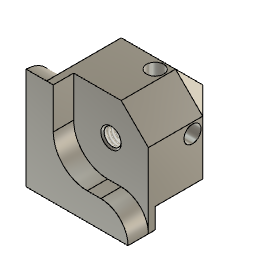
cornerstone-a (Autodesk Fusion 360 design; units mm, degrees)
Autodesk Fusion 360 part; units mm, degrees
sketch "Sketch1" plane through (0, 0, 0) normal (0, 0, 1) x (1, 0, 0)
  line L0 (0, 0) -> (15, 0)
  line L1 (15, 0) -> (15, 15)
  line L2 (15, 15) -> (0, 15)
  line L3 (0, 15) -> (0, 0)
  dimension "d5" = 15
  dimension "d6" = 15
  constraint horizontal L0
  constraint vertical L1
  constraint horizontal L2
  constraint vertical L3
  constraint coincident L0.start L3.end
  measures "d5" distance of L0.start L0.end
  measures "d6" distance of L0.start L2.end
extrude "Extrude1" add sketch "Sketch1" along normal blind 15
sketch "Sketch2" plane through (0, 0, 0) normal (0, -1, 0) x (1, 0, 0)
  line L0 (0, 0) -> (15, 0)
  line L1 (15, 0) -> (15, 15)
  line L2 (15, 15) -> (0, 15)
  line L3 (0, 15) -> (0, 0)
  line L4 (4, 4) -> (15, 4)
  line L5 (15, 4) -> (15, 15)
  line L6 (15, 15) -> (4, 15)
  line L7 (4, 15) -> (4, 4)
  point P0 (4, 4)
  dimension "d9" = 4
  dimension "d10" = 4
  constraint horizontal L4
  constraint vertical L5
  constraint horizontal L6
  constraint vertical L7
  constraint coincident L1.end L2.start
  constraint coincident P0 L4.start
  measures "d9" distance of L3 P0
  measures "d10" distance of L0 P0
extrude "Extrude2" cut sketch "Sketch2" against normal blind 3 contours L1 L2 L4 L5 L6 L7
sketch "Sketch3" plane through (0, 0, 0) normal (-1, 0, 0) x (0, -1, 0)
  line L0 (-15, 0) -> (0, 0)
  line L1 (0, 0) -> (0, 15)
  line L2 (0, 15) -> (-15, 15)
  line L3 (-15, 15) -> (-15, 0)
  line L4 (-4, 4) -> (-15, 4)
  line L5 (-15, 4) -> (-15, 15)
  line L6 (-15, 15) -> (-4, 15)
  line L7 (-4, 15) -> (-4, 4)
  point P0 (-4, 4)
  dimension "d14" = 4
  dimension "d15" = 4
  constraint horizontal L4
  constraint vertical L5
  constraint horizontal L6
  constraint vertical L7
  constraint coincident L2.end L3.start
  constraint coincident P0 L4.start
  measures "d14" distance of L1 P0
  measures "d15" distance of L0 P0
extrude "Extrude3" cut sketch "Sketch3" against normal blind 3 contours L2 L3 L4 L5 L6 L7
sketch "Sketch4" plane through (0, 0, 0) normal (0, 0, -1) x (1, 0, 0)
  line L0 (0, 0) -> (0, -15)
  line L1 (0, -15) -> (15, -15)
  line L2 (15, -15) -> (15, 0)
  line L3 (15, 0) -> (0, 0)
  line L4 (4, -4) -> (15, -4)
  line L5 (15, -4) -> (15, -15)
  line L6 (15, -15) -> (4, -15)
  line L7 (4, -15) -> (4, -4)
  point P0 (4, -4)
  dimension "d18" = 4
  dimension "d19" = 4
  constraint horizontal L4
  constraint vertical L5
  constraint horizontal L6
  constraint vertical L7
  constraint coincident L1.end L2.start
  constraint coincident P0 L4.start
  measures "d18" distance of L0 P0
  measures "d19" distance of L3 P0
extrude "Extrude4" cut sketch "Sketch4" against normal blind 3 contours L1 L2 L4 L5 L6 L7
sketch "Sketch5" plane through (0, 3, 0) normal (0, -1, 0) x (1, 0, 0)
  line L0 (4, 15) -> (4, 4)
  line L1 (4, 4) -> (15, 4)
  line L2 (15, 4) -> (15, 15)
  line L3 (15, 15) -> (4, 15)
  point P0 (9.5, 9.5)
  dimension "d42" = 5.5
  dimension "d43" = 5.5
  measures "d42" horizontal distance of L0.end P0
  measures "d43" vertical distance of L0.end P0
sketch "Sketch6" plane through (3, 0, 0) normal (-1, 0, 0) x (0, -1, 0)
  line L0 (-4, 15) -> (-15, 15)
  line L1 (-15, 15) -> (-15, 4)
  line L2 (-15, 4) -> (-4, 4)
  line L3 (-4, 4) -> (-4, 15)
  point P0 (-9.5, 9.5)
  dimension "d44" = 5.5
  dimension "d45" = 5.5
  measures "d44" horizontal distance of L2.end P0
  measures "d45" vertical distance of L2.end P0
sketch "Sketch7" plane through (0, 0, 3) normal (0, 0, -1) x (1, 0, 0)
  line L0 (4, -15) -> (15, -15)
  line L1 (15, -15) -> (15, -4)
  line L2 (15, -4) -> (4, -4)
  line L3 (4, -4) -> (4, -15)
  point P0 (9.5, -9.5)
  dimension "d46" = 5.5
  dimension "d47" = 5.5
  measures "d46" horizontal distance of L2.end P0
  measures "d47" vertical distance of L2.end P0
hole "Hole4" at (9.5, 3, 9.5) direction (0, 1, 0) diameter 2.529 end through all countersink diameter 3 countersink angle 90
thread "Thread4" "ISO Metric profile 3.0 M3x0.5 6H" thread offset 0 thread depth 5
hole "Hole5" at (3, 9.5, 9.5) direction (1, 0, 0) diameter 2.529 end through all countersink diameter 3 countersink angle 90
thread "Thread5" "ISO Metric profile 3.0 M3x0.5 6H" thread offset 0 thread depth 5
hole "Hole6" at (9.5, 9.5, 3) direction (0, 0, 1) diameter 2.529 end through all countersink diameter 3 countersink angle 90
thread "Thread6" "ISO Metric profile 3.0 M3x0.5 6H" thread offset 0 thread depth 5
fillet "Fillet3" radius 5 3 edges at (4, 1.5, 4) (1.5, 4, 4) (4, 4, 1.5)
chamfer "Chamfer2" distance 4 angle 45 3 edges at (15, 9, 15) (15, 15, 9) (9, 15, 15)
fillet "Fillet4" radius 4 3 edges at (1.5, 4, 15) (15, 1.5, 4) (4, 15, 1.5)
equation "length_rib = 15 mm"
equation "distance_corner = 4 mm"
equation "distance_remaining = length_rib - distance_corner"
equation "distance_hole = distance_remaining / 2"
equation "d5 = length_rib"
equation "d6 = length_rib"
equation "d7 = length_rib"
equation "d9 = distance_corner"
equation "d10 = distance_corner"
equation "plate_thickness = 3 mm"
equation "d12 = -plate_thickness"
equation "d14 = distance_corner"
equation "d15 = distance_corner"
equation "d16 = -plate_thickness"
equation "d18 = distance_corner"
equation "d19 = distance_corner"
equation "d20 = -plate_thickness"
equation "d42 = distance_remaining / 2"
equation "d43 = distance_remaining / 2"
equation "d44 = distance_remaining / 2"
equation "d45 = distance_remaining / 2"
equation "d46 = distance_remaining / 2"
equation "d47 = distance_remaining / 2"
